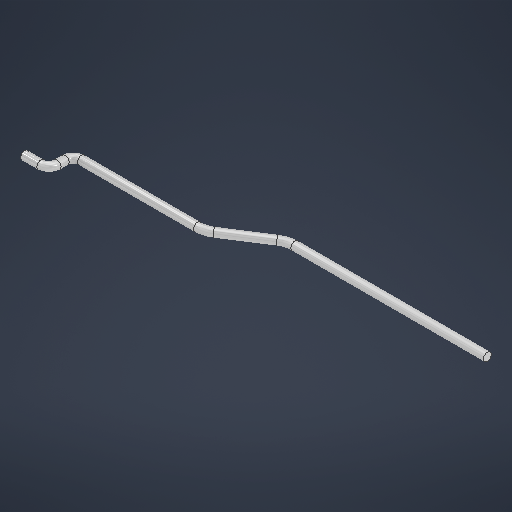
# Autodesk Inventor part: P_aft_servolink
Saved by Autodesk Inventor 2026 (Build 300175000, 175)
## iProperties
Created: 2025-09-02
Part Number: P_aft_servolink
Material: Generisch
Document SubType Name: Modeling
Designer: FAL
Density: 1 g/cm^3
Appearance: Vorgabe
Author: FAL
Autodesk Inventor part; units mm, degrees
ref_plane "YZ Plane" through (0, 0, 0) normal (1, 0, 0) x (0, 1, 0)
ref_plane "XZ Plane" through (0, 0, 0) normal (0, 1, 0) x (-1, 0, 0)
ref_plane "XY Plane" through (0, 0, 0) normal (0, 0, 1) x (1, 0, 0)
sketch "Skizze1" plane through (0, 0, 0) normal (0, 0, 1) x (1, 0, 0)
  line L0 (0, 0) -> (2, 0)
  line L1 (3, 1) -> (3, 2)
  arc A0 (2, 0) -> (3, 1) centre (2, 1) ccw
  arc A1 (4, 3) -> (3, 2) centre (4, 2) ccw
  line L2 (4, 3) -> (18.2842, 3)
  line L3 (19.9027, 3.4741) -> (24.6657, 6.5259)
  line L4 (26.2842, 7) -> (50, 7)
  arc A2 (18.2842, 3) -> (19.9027, 3.4741) centre (18.2842, 6) ccw
  arc A3 (26.2842, 7) -> (24.6657, 6.5259) centre (26.2842, 4) ccw
  dimension "d0" = 1
  dimension "d4" = 2
  dimension "d9" = 3
  dimension "d10" = 4
  dimension "d11" = 50
  dimension "d12" = 3
  dimension "d13" = 8
  constraints: 10 end point, 8 point on circle, 8 tangent, 4 centre point, 2 equal radius, 2 horizontal, 2 perpendicular
  measures "d0" radius of A0
  measures "d4" horizontal distance of L0.start A0.centre
  measures "d9" radius of A2
  measures "d10" distance between parallel lines of L2 L4
  measures "d11" horizontal distance of L0.start L4.end
  measures "d12" distance from line of L0.start L2
  measures "d13" horizontal distance of A3.centre A2.centre
sketch "Skizze2" plane through (0, 0, 0) normal (1, 0, 0) x (0, 1, 0)
  circle A0 centre (0, 0) radius 0.5
  dimension "d1" = 1
  constraints: 1 centre point, 1 coincident
  measures "d1" diameter of A0
sweep "Sweeping1" add profiles "Skizze2" path "Skizze1" path curves L0 A0 L1 A1 L2 A2 L3 A3 L4
